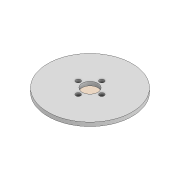
# Autodesk Inventor part: 2_75 in spool inner plate
Saved by Autodesk Inventor 2020 (Build 240168000, 168)
## iProperties
Created: 2017-11-20
Part Number: 2_75 in spool inner plate
Material: Generic
Document SubType Name: Modeling
Designer: ball
Density: 1 g/cm^3
Appearance: Default
Author: ball
Revision Number: ANY
Autodesk Inventor part; units mm, degrees
ref_plane "YZ Plane" through (0, 0, 0) normal (1, 0, 0) x (0, 1, 0)
ref_plane "XZ Plane" through (0, 0, 0) normal (0, 1, 0) x (-1, 0, 0)
ref_plane "XY Plane" through (0, 0, 0) normal (0, 0, 1) x (1, 0, 0)
ref_plane "Work Plane1" through (0, 1.5875, 0) normal (0, 1, 0) x (1, 0, 0)
sketch "Sketch1" plane through (0, 1.5875, 0) normal (0, 1, 0) x (1, 0, 0)
  circle A0 centre (0, 0) radius 34.925
  circle A1 centre (0, -9.779) radius 1.778 construction
  circle A2 centre (-9.779, 0) radius 1.778 construction
  circle A3 centre (0, 9.779) radius 1.778 construction
  circle A4 centre (9.779, 0) radius 1.778 construction
  circle A5 centre (0, 0) radius 6.35 construction
  circle A6 centre (0, -9.779) radius 1.9304
  circle A7 centre (-9.779, 0) radius 1.9304
  circle A8 centre (0, 9.779) radius 1.9304
  circle A9 centre (9.779, 0) radius 1.9304
  circle A10 centre (0, 0) radius 6.477
  line L0 (0, 0) -> (44.45, 0) construction
  dimension "d1" = 69.85
  dimension "d2" = 3.8608
  dimension "d3" = 3.8608
  dimension "d5" = 3.8608
  dimension "d6" = 12.954
  constraints: 7 coincident, 6 centre point, 2 end point, 1 horizontal
  measures "d1" diameter of A0
  measures "d2" diameter of A6
  measures "d3" diameter of A7
  measures "d5" diameter of A9
  measures "d6" diameter of A10
extrude "Extrusion2" add sketch "Sketch1" along normal blind 3.175
body "Solid3"
